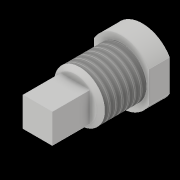
# Autodesk Inventor part: lab10_2
Saved by Autodesk Inventor 2019 (Build 230136000, 136)
## iProperties
Created: 2020-12-02
Part Number: lab10_2
Material: Generic
Document SubType Name: Modeling
Designer: liviu
Density: 1 g/cm^3
Appearance: Default
Author: liviu
Autodesk Inventor part; units mm, degrees
ref_plane "YZ Plane" through (0, 0, 0) normal (1, 0, 0) x (0, 1, 0)
ref_plane "XZ Plane" through (0, 0, 0) normal (0, 1, 0) x (-1, 0, 0)
ref_plane "XY Plane" through (0, 0, 0) normal (0, 0, 1) x (1, 0, 0)
sketch "Sketch1" plane through (0, 0, 0) normal (0, 0, 1) x (1, 0, 0)
  circle A0 centre (0, 0) radius 15
  dimension "d0" = 30
  constraints: 1 centre point, 1 coincident
  measures "d0" diameter of A0
extrude "Extrusion1" add sketch "Sketch1" along normal blind 10
sketch "Sketch2" plane through (0, 0, 10) normal (0, 0, 1) x (1, 0, 0)
  line L0 (-13, -20) -> (13, -20)
  line L1 (13, -20) -> (13, 20)
  line L2 (13, 20) -> (-13, 20)
  line L3 (-13, 20) -> (-13, -20)
  line L4 (-13, -20) -> (13, 20) construction
  line L5 (13, -20) -> (-13, 20) construction
  point P0 (0, 0)
  dimension "d3" = 26
  dimension "d4" = 40
  constraints: 12 end point, 2 midpoint, 2 parallel, 1 horizontal, 1 perpendicular
  measures "d3" distance of L1.end L2.end
  measures "d4" distance of L0.end L1.end
extrude "Extrusion2" cut sketch "Sketch2" against normal blind 10 keep common part
sketch "Sketch3" plane through (0, 0, 10) normal (0, 0, 1) x (1, 0, 0)
  circle A0 centre (0, 0) radius 12
  dimension "d7" = 24
  constraints: 1 centre point, 1 coincident
  measures "d7" diameter of A0
extrude "Extrusion3" add sketch "Sketch3" along normal blind 22
chamfer "Chamfer1" distance 2 angle 45 1 edges at (-12, 0, 32)
sketch "Sketch4" plane through (0, 0, 32) normal (0, 0, 1) x (1, 0, 0)
  line L0 (-7, -7) -> (7, -7)
  line L1 (7, -7) -> (7, 7)
  line L2 (7, 7) -> (-7, 7)
  line L3 (-7, 7) -> (-7, -7)
  line L4 (-7, -7) -> (7, 7) construction
  line L5 (7, -7) -> (-7, 7) construction
  point P0 (0, 0)
  dimension "d13" = 14
  constraints: 12 end point, 2 midpoint, 2 parallel, 2 perpendicular, 1 horizontal
  measures "d13" distance of L1.end L2.end
extrude "Extrusion4" add sketch "Sketch4" along normal blind 18
thread "Thread1" size "TR24x3" class "7e" standard "ISO Metric Trapezoidal Threads" full length
body "Solid1"
